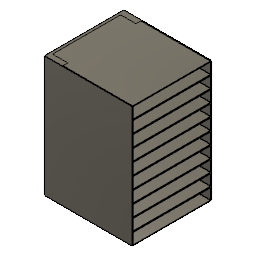
NES Shelf v1 (Autodesk Fusion 360 design; units mm, degrees)
Autodesk Fusion 360 part; units mm, degrees
sketch "Sketch1" plane through (0, 0, 0) normal (1, 0, 0) x (0, 0, -1)
  line L0 (0, 0) -> (120, 0)
  line L1 (120, 0) -> (120, 190)
  line L2 (120, 190) -> (0, 190)
  line L3 (0, 190) -> (0, 0)
  dimension "d2" = 120
  dimension "d3" = 190
  constraint horizontal L0
  constraint vertical L1
  constraint horizontal L2
  constraint vertical L3
  constraint coincident L0.start L3.end
  measures "d2" distance of L0.start L0.end
  measures "d3" distance of L0.start L2.end
extrude "Extrude1" add sketch "Sketch1" along normal blind 134
extrude "Extrude2" add 1 faces at (89.3333, 126.6667, 0) along direction (0, 0, 1) blind 1
extrude "Extrude3" add 1 faces at (89.3333, 63.3333, -120) along direction (0, 0, -1) blind 1
sketch "Sketch2" plane through (134, 0, 0) normal (1, 0, 0) x (0, 0, -1)
  line L0 (-1, 0) -> (121, 0)
  line L1 (121, 0) -> (121, 190)
  line L2 (121, 190) -> (-1, 190)
  line L3 (-1, 190) -> (-1, 0)
  line L4 (60, 190) -> (60, 188.5)
  line L5 (60, 188.5) -> (6.6, 188.5)
  line L6 (6.6, 188.5) -> (6.6, 171)
  line L7 (6.6, 171) -> (113.4, 171)
  line L8 (60, 188.5) -> (113.4, 188.5)
  line L9 (113.4, 188.5) -> (113.4, 171)
  line L10 (6.6, 171) -> (6.6, 169.5)
  line L11 (6.6, 169.5) -> (113.4, 169.5)
  line L12 (113.4, 169.5) -> (113.4, 152)
  line L13 (113.4, 152) -> (6.6, 152)
  line L14 (6.6, 152) -> (6.6, 169.5)
  line L15 (6.6, 152) -> (6.6, 150.5)
  line L16 (6.6, 150.5) -> (113.4, 150.5)
  line L17 (113.4, 150.5) -> (113.4, 133)
  line L18 (113.4, 133) -> (6.6, 133)
  line L19 (6.6, 133) -> (6.6, 150.5)
  line L20 (6.6, 133) -> (6.6, 131.5)
  line L21 (6.6, 131.5) -> (113.4, 131.5)
  line L22 (113.4, 131.5) -> (113.4, 114)
  line L23 (113.4, 114) -> (6.6, 114)
  line L24 (6.6, 114) -> (6.6, 131.5)
  line L25 (6.6, 114) -> (6.6, 112.5)
  line L26 (6.6, 112.5) -> (113.4, 112.5)
  line L27 (113.4, 112.5) -> (113.4, 95)
  line L28 (113.4, 95) -> (6.6, 95)
  line L29 (6.6, 95) -> (6.6, 112.5)
  line L30 (6.6, 95) -> (6.6, 93.5)
  line L31 (6.6, 93.5) -> (113.4, 93.5)
  line L32 (113.4, 93.5) -> (113.4, 76)
  line L33 (113.4, 76) -> (6.6, 76)
  line L34 (6.6, 76) -> (6.6, 93.5)
  line L35 (6.6, 76) -> (6.6, 74.5)
  line L36 (6.6, 74.5) -> (113.4, 74.5)
  line L37 (113.4, 74.5) -> (113.4, 57)
  line L38 (113.4, 57) -> (6.6, 57)
  line L39 (6.6, 57) -> (6.6, 74.5)
  line L40 (6.6, 57) -> (6.6, 55.5)
  line L41 (6.6, 55.5) -> (113.4, 55.5)
  line L42 (113.4, 55.5) -> (113.4, 38)
  line L43 (113.4, 38) -> (6.6, 38)
  line L44 (6.6, 38) -> (6.6, 55.5)
  line L45 (6.6, 38) -> (6.6, 36.5)
  line L46 (6.6, 36.5) -> (113.4, 36.5)
  line L47 (113.4, 36.5) -> (113.4, 19)
  line L48 (113.4, 19) -> (6.6, 19)
  line L49 (6.6, 19) -> (6.6, 36.5)
  line L50 (6.6, 19) -> (6.6, 17.5)
  line L51 (6.6, 17.5) -> (113.4, 17.5)
  line L52 (113.4, 17.5) -> (113.4, 0)
  line L53 (113.4, 0) -> (6.6, 0)
  line L54 (6.6, 0) -> (6.6, 17.5)
  dimension "d10" = 1.5
  dimension "d11" = 53.4
  dimension "d12" = 17.5
  dimension "d13" = 106.8
  dimension "d14" = 53.4
  dimension "d15" = 1.5
  dimension "d16" = 106.8
  dimension "d17" = 17.5
  dimension "d18" = 1.5
  dimension "d19" = 106.8
  dimension "d20" = 17.5
  dimension "d21" = 1.5
  dimension "d22" = 106.8
  dimension "d23" = 17.5
  dimension "d24" = 1.5
  dimension "d25" = 17.5
  dimension "d26" = 106.8
  dimension "d27" = 1.5
  dimension "d28" = 106.8
  dimension "d29" = 17.5
  dimension "d30" = 1.5
  dimension "d31" = 17.5
  dimension "d32" = 106.8
  dimension "d33" = 1.5
  dimension "d34" = 17.5
  dimension "d35" = 106.8
  dimension "d36" = 1.5
  dimension "d37" = 106.8
  dimension "d38" = 17.5
  dimension "d39" = 1.5
  dimension "d40" = 106.8
  dimension "d41" = 17.5
  constraint midpoint L2 L4.start
  constraint perpendicular L7 L9
  constraint horizontal L11
  constraint vertical L12
  constraint horizontal L13
  constraint vertical L14
  constraint horizontal L16
  constraint vertical L17
  constraint horizontal L18
  constraint vertical L19
  constraint horizontal L21
  constraint vertical L22
  constraint horizontal L23
  constraint vertical L24
  constraint horizontal L26
  constraint vertical L27
  constraint horizontal L28
  constraint vertical L29
  constraint horizontal L31
  constraint vertical L32
  constraint horizontal L33
  constraint vertical L34
  constraint horizontal L36
  constraint vertical L37
  constraint horizontal L38
  constraint vertical L39
  constraint horizontal L41
  constraint vertical L42
  constraint horizontal L43
  constraint vertical L44
  constraint horizontal L46
  constraint vertical L47
  constraint horizontal L48
  constraint vertical L49
  constraint horizontal L51
  constraint vertical L52
  constraint horizontal L53
  constraint vertical L54
  measures "d10" distance of L4.start L4.end
  measures "d11" distance of L4.end L5.end
  measures "d12" distance of L5.end L6.end
  measures "d13" distance of L6.end L7.end
  measures "d14" distance of L4.end L8.end
  measures "d15" distance of L6.end L10.end
  measures "d16" distance of L10.end L11.end
  measures "d17" distance of L10.end L13.end
  measures "d18" distance of L13.end L15.end
  measures "d19" distance of L15.end L16.end
  measures "d20" distance of L15.end L18.end
  measures "d21" distance of L18.end L20.end
  measures "d22" distance of L20.end L21.end
  measures "d23" distance of L20.end L23.end
  measures "d24" distance of L23.end L25.end
  measures "d25" distance of L25.end L28.end
  measures "d26" distance of L25.end L26.end
  measures "d27" distance of L28.end L30.end
  measures "d28" distance of L30.end L31.end
  measures "d29" distance of L30.end L33.end
  measures "d30" distance of L33.end L35.end
  measures "d31" distance of L35.end L38.end
  measures "d32" distance of L35.end L36.end
  measures "d33" distance of L38.end L40.end
  measures "d34" distance of L40.end L43.end
  measures "d35" distance of L40.end L41.end
  measures "d36" distance of L43.end L45.end
  measures "d37" distance of L45.end L46.end
  measures "d38" distance of L45.end L48.end
  measures "d39" distance of L48.end L50.end
  measures "d40" distance of L50.end L51.end
  measures "d41" distance of L50.end L53.end
extrude "Extrude4" add 1 faces at (89.3333, 0, -80.3333) along direction (0, -1, 0) blind 0.75
extrude "Extrude5" cut 1 faces at (89.3333, 190, -80.3333) along direction (0, -1, 0) blind 0.75
extrude "Extrude6" cut sketch "Sketch2" against normal blind 130 contours L0 L51 L52 L53 L54 | L46 L47 L48 L49 | L5 L6 L7 L8 L9 | L41 L42 L43 L44 | L11 L12 L13 L14 | L36 L37 L38 L39 | L16 L17 L18 L19 | L31 L32 L33 L34 | L21 L22 L23 L24 | L26 L27 L28 L29
extrude "Extrude7" add 1 faces at (134, 106.6667, -1.5333) along direction (1, 0, 0) blind 4
sketch "Sketch3" plane through (138, 0, 0) normal (1, 0, 0) x (0, 0, -1)
  line L0 (113.4, 150.5) -> (113.4, 133)
  line L1 (113.4, 133) -> (6.6, 133)
  line L2 (6.6, 133) -> (6.6, 150.5)
  line L3 (6.6, 150.5) -> (113.4, 150.5)
  line L4 (113.4, 74.5) -> (113.4, 57)
  line L5 (113.4, 57) -> (6.6, 57)
  line L6 (6.6, 57) -> (6.6, 74.5)
  line L7 (6.6, 74.5) -> (113.4, 74.5)
  line L8 (113.4, 36.5) -> (113.4, 19)
  line L9 (113.4, 19) -> (6.6, 19)
  line L10 (6.6, 19) -> (6.6, 36.5)
  line L11 (6.6, 36.5) -> (113.4, 36.5)
  line L12 (113.4, 93.5) -> (113.4, 76)
  line L13 (113.4, 76) -> (6.6, 76)
  line L14 (6.6, 76) -> (6.6, 93.5)
  line L15 (6.6, 93.5) -> (113.4, 93.5)
  line L16 (113.4, 169.5) -> (113.4, 152)
  line L17 (113.4, 152) -> (6.6, 152)
  line L18 (6.6, 152) -> (6.6, 169.5)
  line L19 (6.6, 169.5) -> (113.4, 169.5)
  line L20 (113.4, 131.5) -> (113.4, 114)
  line L21 (113.4, 114) -> (6.6, 114)
  line L22 (6.6, 114) -> (6.6, 131.5)
  line L23 (6.6, 131.5) -> (113.4, 131.5)
  line L24 (113.4, 55.5) -> (113.4, 38)
  line L25 (113.4, 38) -> (6.6, 38)
  line L26 (6.6, 38) -> (6.6, 55.5)
  line L27 (6.6, 55.5) -> (113.4, 55.5)
  line L28 (113.4, 17.5) -> (113.4, 0)
  line L29 (113.4, 0) -> (6.6, 0)
  line L30 (6.6, 0) -> (6.6, 17.5)
  line L31 (6.6, 17.5) -> (113.4, 17.5)
  line L32 (113.4, 112.5) -> (113.4, 95)
  line L33 (113.4, 95) -> (6.6, 95)
  line L34 (6.6, 95) -> (6.6, 112.5)
  line L35 (6.6, 112.5) -> (113.4, 112.5)
  line L36 (6.6, 171) -> (6.6, 188.5)
  line L37 (6.6, 188.5) -> (113.4, 188.5)
  line L38 (113.4, 188.5) -> (113.4, 171)
  line L39 (113.4, 171) -> (6.6, 171)
  line L40 (121, 189.25) -> (-1, 189.25)
  line L41 (-1, 189.25) -> (-1, -0.75)
  line L42 (-1, -0.75) -> (121, -0.75)
  line L43 (121, -0.75) -> (121, 189.25)
  line L44 (6.6, 188.5) -> (-0.9, 188.5)
  line L45 (-0.9, 188.5) -> (-0.9, 171)
  line L46 (-0.9, 171) -> (6.6, 171)
  line L47 (6.6, 171) -> (6.6, 188.5)
  line L48 (113.4, 188.5) -> (120.9, 188.5)
  line L49 (120.9, 188.5) -> (120.9, 171)
  line L50 (120.9, 171) -> (113.4, 171)
  line L51 (113.4, 171) -> (113.4, 188.5)
  line L52 (113.4, 169.5) -> (120.9, 169.5)
  line L53 (120.9, 169.5) -> (120.9, 152)
  line L54 (120.9, 152) -> (113.4, 152)
  line L55 (113.4, 152) -> (113.4, 169.5)
  line L56 (113.4, 133) -> (120.9, 133)
  line L57 (120.9, 133) -> (120.9, 150.5)
  line L58 (120.9, 150.5) -> (113.4, 150.5)
  line L59 (113.4, 150.5) -> (113.4, 133)
  line L60 (113.4, 131.5) -> (120.9, 131.5)
  line L61 (120.9, 131.5) -> (120.9, 114)
  line L62 (120.9, 114) -> (113.4, 114)
  line L63 (113.4, 114) -> (113.4, 131.5)
  line L64 (113.4, 112.5) -> (120.9, 112.5)
  line L65 (120.9, 112.5) -> (120.9, 95)
  line L66 (120.9, 95) -> (113.4, 95)
  line L67 (113.4, 95) -> (113.4, 112.5)
  line L68 (113.4, 93.5) -> (120.9, 93.5)
  line L69 (120.9, 93.5) -> (120.9, 76)
  line L70 (120.9, 76) -> (113.4, 76)
  line L71 (113.4, 76) -> (113.4, 93.5)
  line L72 (113.4, 74.5) -> (120.9, 74.5)
  line L73 (120.9, 74.5) -> (120.9, 57)
  line L74 (120.9, 57) -> (113.4, 57)
  line L75 (113.4, 57) -> (113.4, 74.5)
  line L76 (113.4, 55.5) -> (120.9, 55.5)
  line L77 (120.9, 55.5) -> (120.9, 38)
  line L78 (120.9, 38) -> (113.4, 38)
  line L79 (113.4, 38) -> (113.4, 55.5)
  line L80 (113.4, 36.5) -> (120.9, 36.5)
  line L81 (120.9, 36.5) -> (120.9, 19)
  line L82 (120.9, 19) -> (113.4, 19)
  line L83 (113.4, 19) -> (113.4, 36.5)
  line L84 (113.4, 17.5) -> (120.9, 17.5)
  line L85 (120.9, 17.5) -> (120.9, 0)
  line L86 (120.9, 0) -> (113.4, 0)
  line L87 (113.4, 0) -> (113.4, 17.5)
  line L88 (6.6, 0) -> (-0.9, 0)
  line L89 (-0.9, 0) -> (-0.9, 17.5)
  line L90 (-0.9, 17.5) -> (6.6, 17.5)
  line L91 (6.6, 17.5) -> (6.6, 0)
  line L92 (6.6, 19) -> (-0.9, 19)
  line L93 (-0.9, 19) -> (-0.9, 36.5)
  line L94 (-0.9, 36.5) -> (6.6, 36.5)
  line L95 (6.6, 36.5) -> (6.6, 19)
  line L96 (6.6, 38) -> (-0.9, 38)
  line L97 (-0.9, 38) -> (-0.9, 55.5)
  line L98 (-0.9, 55.5) -> (6.6, 55.5)
  line L99 (6.6, 55.5) -> (6.6, 38)
  line L100 (6.6, 57) -> (-0.9, 57)
  line L101 (-0.9, 57) -> (-0.9, 74.5)
  line L102 (-0.9, 74.5) -> (6.6, 74.5)
  line L103 (6.6, 74.5) -> (6.6, 57)
  line L104 (6.6, 76) -> (-0.9, 76)
  line L105 (-0.9, 76) -> (-0.9, 93.5)
  line L106 (-0.9, 93.5) -> (6.6, 93.5)
  line L107 (6.6, 93.5) -> (6.6, 76)
  line L108 (6.6, 95) -> (-0.9, 95)
  line L109 (-0.9, 95) -> (-0.9, 112.5)
  line L110 (-0.9, 112.5) -> (6.6, 112.5)
  line L111 (6.6, 112.5) -> (6.6, 95)
  line L112 (6.6, 114) -> (-0.9, 114)
  line L113 (-0.9, 114) -> (-0.9, 131.5)
  line L114 (-0.9, 131.5) -> (6.6, 131.5)
  line L115 (6.6, 131.5) -> (6.6, 114)
  line L116 (6.6, 133) -> (-0.9, 133)
  line L117 (-0.9, 133) -> (-0.9, 150.5)
  line L118 (-0.9, 150.5) -> (6.6, 150.5)
  line L119 (6.6, 150.5) -> (6.6, 133)
  line L120 (6.6, 152) -> (-0.9, 152)
  line L121 (-0.9, 152) -> (-0.9, 169.5)
  line L122 (-0.9, 169.5) -> (6.6, 169.5)
  line L123 (6.6, 169.5) -> (6.6, 152)
  dimension "d54" = 7.5
  dimension "d55" = 17.5
  dimension "d56" = 7.5
  dimension "d57" = 17.5
  dimension "d58" = 7.5
  dimension "d59" = 7.5
  dimension "d60" = 7.5
  dimension "d61" = 17.5
  dimension "d62" = 7.5
  dimension "d63" = 17.5
  dimension "d64" = 7.5
  dimension "d65" = 17.5
  dimension "d66" = 7.5
  dimension "d67" = 7.5
  dimension "d68" = 17.5
  dimension "d69" = 7.5
  dimension "d70" = 7.5
  dimension "d71" = 17.5
  dimension "d72" = 17.5
  dimension "d73" = 7.5
  dimension "d74" = 17.5
  dimension "d75" = 7.5
  dimension "d76" = 17.5
  dimension "d77" = 7.5
  dimension "d78" = 17.5
  dimension "d79" = 7.5
  dimension "d80" = 7.5
  dimension "d81" = 17.5
  dimension "d82" = 17.5
  dimension "d83" = 7.5
  dimension "d84" = 7.5
  dimension "d85" = 17.5
  dimension "d86" = 7.5
  dimension "d87" = 17.5
  dimension "d88" = 17.5
  dimension "d89" = 7.5
  constraint horizontal L44
  constraint vertical L45
  constraint horizontal L46
  constraint vertical L47
  constraint coincident L36.end L37.start
  constraint horizontal L48
  constraint vertical L49
  constraint horizontal L50
  constraint vertical L51
  constraint coincident L37.end L38.start
  constraint horizontal L52
  constraint vertical L53
  constraint horizontal L54
  constraint vertical L55
  constraint coincident L16.start L19.end
  constraint horizontal L56
  constraint vertical L57
  constraint horizontal L58
  constraint vertical L59
  constraint coincident L0.end L1.start
  constraint horizontal L60
  constraint vertical L61
  constraint horizontal L62
  constraint vertical L63
  constraint coincident L20.start L23.end
  constraint horizontal L64
  constraint vertical L65
  constraint horizontal L66
  constraint vertical L67
  constraint coincident L32.start L35.end
  constraint horizontal L68
  constraint vertical L69
  constraint horizontal L70
  constraint vertical L71
  constraint coincident L12.start L15.end
  constraint horizontal L72
  constraint vertical L73
  constraint horizontal L74
  constraint vertical L75
  constraint coincident L4.start L7.end
  constraint horizontal L76
  constraint vertical L77
  constraint horizontal L78
  constraint vertical L79
  constraint coincident L24.start L27.end
  constraint horizontal L80
  constraint vertical L81
  constraint horizontal L82
  constraint vertical L83
  constraint coincident L8.start L11.end
  constraint horizontal L84
  constraint vertical L85
  constraint horizontal L86
  constraint vertical L87
  constraint coincident L28.start L31.end
  constraint horizontal L88
  constraint vertical L89
  constraint horizontal L90
  constraint vertical L91
  constraint coincident L29.end L30.start
  constraint horizontal L92
  constraint vertical L93
  constraint horizontal L94
  constraint vertical L95
  constraint coincident L9.end L10.start
  constraint horizontal L96
  constraint vertical L97
  constraint horizontal L98
  constraint vertical L99
  constraint coincident L25.end L26.start
  constraint horizontal L100
  constraint vertical L101
  constraint horizontal L102
  constraint vertical L103
  constraint coincident L5.end L6.start
  constraint horizontal L104
  constraint vertical L105
  constraint horizontal L106
  constraint vertical L107
  constraint coincident L13.end L14.start
  constraint horizontal L108
  constraint vertical L109
  constraint horizontal L110
  constraint vertical L111
  constraint coincident L33.end L34.start
  constraint horizontal L112
  constraint vertical L113
  constraint horizontal L114
  constraint vertical L115
  constraint coincident L21.end L22.start
  constraint horizontal L116
  constraint vertical L117
  constraint horizontal L118
  constraint vertical L119
  constraint coincident L1.end L2.start
  constraint horizontal L120
  constraint vertical L121
  constraint horizontal L122
  constraint vertical L123
  constraint coincident L17.end L18.start
  measures "d54" distance of L36.end L44.end
  measures "d55" distance of L37.end L38.end
  measures "d56" distance of L37.end L48.end
  measures "d57" distance of L16.start L16.end
  measures "d58" distance of L16.start L52.end
  measures "d59" distance of L0.end L56.end
  measures "d60" distance of L20.start L60.end
  measures "d61" distance of L32.start L32.end
  measures "d62" distance of L32.start L64.end
  measures "d63" distance of L12.start L12.end
  measures "d64" distance of L12.start L68.end
  measures "d65" distance of L4.start L4.end
  measures "d66" distance of L4.start L72.end
  measures "d67" distance of L24.start L76.end
  measures "d68" distance of L8.start L8.end
  measures "d69" distance of L8.start L80.end
  measures "d70" distance of L28.start L84.end
  measures "d71" distance of L28.start L28.end
  measures "d72" distance of L29.end L30.end
  measures "d73" distance of L29.end L88.end
  measures "d74" distance of L9.end L10.end
  measures "d75" distance of L9.end L92.end
  measures "d76" distance of L25.end L26.end
  measures "d77" distance of L25.end L96.end
  measures "d78" distance of L5.end L6.end
  measures "d79" distance of L5.end L100.end
  measures "d80" distance of L13.end L104.end
  measures "d81" distance of L13.end L14.end
  measures "d82" distance of L33.end L34.end
  measures "d83" distance of L33.end L108.end
  measures "d84" distance of L21.end L112.end
  measures "d85" distance of L21.end L22.end
  measures "d86" distance of L1.end L116.end
  measures "d87" distance of L1.end L2.end
  measures "d88" distance of L17.end L18.end
  measures "d89" distance of L17.end L120.end
extrude "Extrude10" cut sketch "Sketch3" against normal blind 110 contours L0 L56 L57 L58 L59 | L2 L116 L117 L118 L119 | L4 L72 L73 L74 L75 | L6 L100 L101 L102 L103 | L8 L80 L81 L82 L83 | L10 L92 L93 L94 L95 | L12 L68 L69 L70 L71 | L14 L104 L105 L106 L107 | L16 L52 L53 L54 L55 | L18 L120 L121 L122 L123 | L20 L60 L61 L62 L63 | L22 L112 L113 L114 L115 | L24 L76 L77 L78 L79 | L26 L96 L97 L98 L99 | L28 L84 L85 L86 L87 | L30 L88 L89 L90 L91 | L32 L64 L65 L66 L67 | L34 L108 L109 L110 L111 | L36 L44 L45 L46 L47 | L38 L48 L49 L50 L51
extrude "Extrude8" add 1 faces at (92, 62.5833, -121) along direction (0, 0, -1) blind 1
extrude "Extrude9" add 1 faces at (92, 62.5833, 1) along direction (0, 0, 1) blind 1
extrude "Extrude11" add 1 faces at (92, 62.5833, -122) along direction (0, 0, -1) blind 0.4
extrude "Extrude12" add 1 faces at (92, 62.5833, 2) along direction (0, 0, 1) blind 0.4
